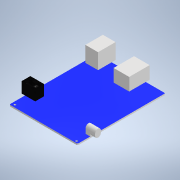
# Autodesk Inventor part: Stemboard
Saved by Autodesk Inventor 2022 (Build 260153000, 153)
## iProperties
Created: 2025-06-23
Part Number: Stemboard
Material: Типовые
Document SubType Name: Modeling
Designer: korsh524
Density: 1 g/cm^3
Appearance: По умолчанию
Author: korsh524
Autodesk Inventor part; units mm, degrees
ref_plane "YZ Plane" through (0, 0, 0) normal (1, 0, 0) x (0, 1, 0)
ref_plane "XZ Plane" through (0, 0, 0) normal (0, 1, 0) x (-1, 0, 0)
ref_plane "XY Plane" through (0, 0, 0) normal (0, 0, 1) x (1, 0, 0)
sketch "Эскиз1" plane through (0, 0, 0) normal (0, 1, 0) x (-1, 0, 0)
  line L0 (0, 0) -> (70, 0)
  line L1 (70, 0) -> (70, 90)
  line L2 (70, 90) -> (0, 90)
  line L3 (0, 90) -> (0, 0)
  dimension "d0" = 70
  dimension "d1" = 90
  constraints: 8 end point, 2 parallel, 1 horizontal, 1 perpendicular
  measures "d0" distance of L2.end L1.end
  measures "d1" distance of L1.end L0.end
extrude "Выдавливание1" add sketch "Эскиз1" along normal blind 1.5
fillet "Сопряжение1" radius 1 4 edges at (0, 0.75, 90) (0, 0.75, 0) (-70, 0.75, 90) (-70, 0.75, 0)
sketch "Эскиз2" plane through (0, 1.5, 0) normal (0, 1, 0) x (1, 0, 0)
  line L0 (-59.5, -74) -> (-73.5, -74)
  line L1 (-73.5, -74) -> (-73.5, -65)
  line L2 (-73.5, -65) -> (-59.5, -65)
  line L3 (-59.5, -65) -> (-59.5, -74)
  line L4 (-69, -90) -> (-1, -90) projected
  line L5 (-70, -1) -> (-70, -89) projected
  point P0 (0, 0)
  dimension "d5" = 16
  dimension "d6" = 9
  dimension "d7" = 14
  dimension "d8" = 3.5
  constraints: 8 end point, 2 parallel, 1 horizontal, 1 perpendicular
  measures "d5" distance between parallel lines of L0 L4
  measures "d6" distance of L0.end L1.end
  measures "d7" distance of L1.end L2.end
  measures "d8" distance between parallel lines of L1 L5
extrude "Выдавливание2" add sketch "Эскиз2" along normal blind 11
sketch "Эскиз3" plane through (0, 1.5, 0) normal (0, 1, 0) x (1, 0, 0)
  line L0 (5, -77) -> (-4.77, -77)
  line L1 (-4.77, -77) -> (-4.77, -71)
  line L2 (-4.77, -71) -> (5, -71)
  line L3 (5, -71) -> (5, -77)
  line L4 (-69, -90) -> (-1, -90) projected
  line L5 (0, -89) -> (0, -1) projected
  point P0 (0, 0)
  dimension "d11" = 6
  dimension "d12" = 13
  dimension "d13" = 5
  constraints: 8 end point, 2 parallel, 1 horizontal, 1 perpendicular
  measures "d11" distance of L0.end L1.end
  measures "d12" distance between parallel lines of L0 L4
  measures "d13" distance between parallel lines of L5 L3
extrude "Выдавливание3" add sketch "Эскиз3" along normal blind 8
fillet "Сопряжение2" radius 3 4 edges at (0.115, 9.5, 71) (0.115, 9.5, 77) (2.5, 1.5, 77) (2.5, 1.5, 71)
sketch "Эскиз4" plane through (0, 1.5, 0) normal (0, 1, 0) x (1, 0, 0)
  line L0 (-20, -17) -> (-36, -17)
  line L1 (-36, -17) -> (-36, 4)
  line L2 (-36, 4) -> (-20, 4)
  line L3 (-20, 4) -> (-20, -17)
  line L4 (-1, 0) -> (-69, 0) projected
  line L5 (0, -71) -> (0, -1) projected
  point P0 (0, 0)
  dimension "d17" = 21
  dimension "d18" = 16
  dimension "d19" = 4
  dimension "d20" = 20
  constraints: 8 end point, 2 parallel, 1 horizontal, 1 perpendicular
  measures "d17" distance of L2.end L0.start
  measures "d18" distance of L1.end L2.end
  measures "d19" distance between parallel lines of L4 L2
  measures "d20" distance between parallel lines of L5 L3
extrude "Выдавливание4" add sketch "Эскиз4" along normal blind 13
sketch "Эскиз5" plane through (0, 1.5, 0) normal (0, 1, 0) x (1, 0, 0)
  line L0 (-55, -14) -> (-68, -14)
  line L1 (-68, -14) -> (-68, 4)
  line L2 (-68, 4) -> (-55, 4)
  line L3 (-55, 4) -> (-55, -14)
  line L4 (-70, -1) -> (-70, -65) projected
  line L5 (-36, 0) -> (-69, 0) projected
  point P0 (0, 0)
  dimension "d23" = 18
  dimension "d24" = 13
  dimension "d25" = 2
  dimension "d26" = 4
  constraints: 8 end point, 2 parallel, 1 horizontal, 1 perpendicular
  measures "d23" distance of L0.end L1.end
  measures "d24" distance between parallel lines of L1 L3
  measures "d25" distance between parallel lines of L1 L4
  measures "d26" distance between parallel lines of L5 L2
extrude "Выдавливание5" add sketch "Эскиз5" along normal blind 16
sketch "Эскиз6" plane through (0, 1.5, 0) normal (0, 1, 0) x (1, 0, 0)
  arc A0 (-1, -90) -> (0, -89) centre (-1, -89) ccw projected
  arc A1 (-70, -89) -> (-69, -90) centre (-69, -89) ccw projected
  circle A2 centre (-67, -87.4129) radius 1
  line L0 (-68, -14) -> (-68, 0) projected
  line L1 (-68, 0) -> (-69, 0) projected
  arc A3 (-69, 0) -> (-70, -1) centre (-69, -1) ccw projected
  line L2 (-70, -1) -> (-70, -65) projected
  line L3 (-70, -65) -> (-59.5, -65) projected
  line L4 (-59.5, -65) -> (-59.5, -74) projected
  line L5 (-59.5, -74) -> (-70, -74) projected
  line L6 (-70, -74) -> (-70, -89) projected
  arc A4 (-70, -89) -> (-69, -90) centre (-69, -89) ccw projected
  line L7 (-69, -90) -> (-1, -90) projected
  arc A5 (-1, -90) -> (0, -89) centre (-1, -89) ccw projected
  line L8 (0, -89) -> (0, -77) projected
  line L9 (0, -77) -> (-4.77, -77) projected
  line L10 (-4.77, -77) -> (-4.77, -71) projected
  line L11 (-4.77, -71) -> (0, -71) projected
  line L12 (0, -71) -> (0, -1) projected
  arc A6 (0, -1) -> (-1, 0) centre (-1, -1) ccw projected
  line L13 (-1, 0) -> (-20, 0) projected
  line L14 (-20, 0) -> (-20, -17) projected
  line L15 (-20, -17) -> (-36, -17) projected
  line L16 (-36, -17) -> (-36, 0) projected
  line L17 (-36, 0) -> (-55, 0) projected
  line L18 (-55, 0) -> (-55, -14) projected
  line L19 (-55, -14) -> (-68, -14) projected
  circle A7 centre (-3, -88) radius 1
  point P0 (0, 0)
  dimension "d29" = 2
  dimension "d30" = 2
  dimension "d31" = 64
  dimension "d32" = 70
  dimension "d33" = 3
  constraints: 2 centre point
  measures "d29" diameter of A2
  measures "d30" distance from line of L7 A7.centre
  measures "d31" horizontal distance of A2.centre A7.centre
  measures "d32" distance between parallel lines of L8 L6
  measures "d33" distance from line of A2.centre L6
extrude "Выдавливание6" cut sketch "Эскиз6" against normal blind 3 contours A2 | A7
equation "\"d34\" = d33"
